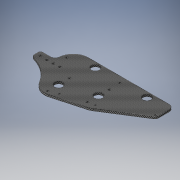
# Autodesk Inventor part: Flywheel Bracket 1
Saved by Autodesk Inventor 2019.4 (Build 234330000, 330)
## iProperties
Created: 2020-01-06
Part Number: Flywheel Bracket 1
Material: CFRP
Document SubType Name: Modeling
Designer: admin
Density: 1.43 g/cm^3
Appearance: Carbon Fiber
Mass: 143.228 g
Surface Area: 462.815 cm^2
Volume: 100.16 cm^3
Author: admin
Autodesk Inventor part; units mm, degrees
ref_plane "YZ Plane" through (0, 0, 0) normal (1, 0, 0) x (0, 1, 0)
ref_plane "XZ Plane" through (0, 0, 0) normal (0, 1, 0) x (-1, 0, 0)
ref_plane "XY Plane" through (0, 0, 0) normal (0, 0, 1) x (1, 0, 0)
sketch "Sketch1" plane through (0, 0, 0) normal (0, 1, 0) x (-1, 0, 0)
  circle A0 centre (-15.2408, 30.085) radius 9.5
  circle A1 centre (-15.2408, 30.085) radius 41.275 construction
  circle A2 centre (44.7592, 83) radius 9.5
  circle A3 centre (113.125, 107.1321) radius 9.5
  circle A4 centre (104.7592, 30.085) radius 9.5
  circle A5 centre (104.7592, 30.085) radius 41.275 construction
  line L0 (104.7592, 30.085) -> (-15.2408, 30.085) construction
  circle A6 centre (44.7592, 83) radius 32.5 construction
  circle A7 centre (113.125, 107.1321) radius 32.5 construction
  circle A8 centre (44.7592, -74.69) radius 88.9 construction
  line L1 (144.134, -74.69) -> (-106.866, -74.69) construction
  line L2 (113.125, 107.1321) -> (44.7592, 83) construction
  line L3 (44.7592, 83) -> (-15.2408, 30.085) construction
  line L4 (113.125, 107.1321) -> (104.7592, 30.085) construction
  line L5 (44.7592, 83) -> (104.7592, 30.085) construction
  line L6 (44.7592, 30.085) -> (44.7592, -74.69) construction
  line L7 (168.125, 18.085) -> (-65.2408, 18.085)
  line L8 (-65.2408, 18.085) -> (-65.2408, 58.085)
  line L9 (-65.2408, 58.085) -> (29.4431, 117.669)
  line L10 (29.4431, 117.669) -> (127.8623, 144.9403)
  line L11 (127.8623, 144.9403) -> (168.125, 80.31)
  line L12 (168.125, 80.31) -> (202.259, 80.31)
  line L13 (202.259, 80.31) -> (202.259, 60.31)
  line L14 (168.125, 18.085) -> (168.125, 60.31)
  line L15 (168.125, 60.31) -> (202.259, 60.31)
  line L16 (168.125, 80.31) -> (168.125, 60.31) construction
  circle A9 centre (44.7592, 83) radius 37.5 construction
  circle A10 centre (192.259, 70.31) radius 2.75
  line L17 (192.259, 70.31) -> (147.259, 70.31) construction
  circle A11 centre (147.259, 70.31) radius 2.75
  circle A12 centre (177.259, 70.31) radius 2.75
  circle A13 centre (162.259, 70.31) radius 2.75
  line L18 (44.7592, 57.6) -> (44.7592, 108.4) construction
  circle A14 centre (44.7592, 57.6) radius 2.75
  circle A15 centre (44.7592, 108.4) radius 2.75
  circle A16 centre (-60.2408, 55.3238) radius 2.2
  circle A17 centre (-60.2408, 55.3238) radius 5 construction
  circle A18 centre (28.7684, 105.4292) radius 2.2
  circle A19 centre (44.7592, 33.085) radius 2.2
  circle A20 centre (93.1857, 124.9549) radius 2.2
  circle A21 centre (158.125, 43.085) radius 2.2
  line L19 (113.125, 81.7321) -> (113.125, 132.5321) construction
  circle A22 centre (113.125, 81.7321) radius 2.75
  circle A23 centre (113.125, 132.5321) radius 2.75
  dimension "d67" = 19
  dimension "d68" = 82.55
  dimension "d69" = 19
  dimension "d70" = 19
  dimension "d71" = 19
  dimension "d72" = 82.55
  dimension "d73" = 65
  dimension "d74" = 65
  dimension "d75" = 120
  dimension "d76" = 177.8
  dimension "d77" = 104.775
  dimension "d78" = 80
  dimension "d79" = 80
  dimension "d80" = 77.5
  dimension "d81" = 72.5
  dimension "d82" = 12
  dimension "d83" = 50
  dimension "d85" = 75
  dimension "d86" = 20
  dimension "d87" = 34.134
  dimension "d88" = 5.5
  dimension "d90" = 5.5
  dimension "d91" = 5.5
  dimension "d93" = 15
  dimension "d95" = 5.5
  dimension "d96" = 15
  dimension "d97" = 15
  dimension "d98" = 10
  dimension "d99" = 10
  dimension "d100" = 135
  dimension "d101" = 40
  dimension "d105" = 55
  dimension "d106" = 50.8
  dimension "d107" = 5.5
  dimension "d108" = 5.5
  dimension "d112" = 4.4
  dimension "d113" = 10
  dimension "d114" = 4.4
  dimension "d115" = 4.4
  dimension "d116" = 4.4
  dimension "d117" = 4.4
  dimension "d118" = 10
  dimension "d119" = 25
  dimension "d120" = 15
  dimension "d121" = 110
  dimension "d122" = 10
  dimension "d123" = 10
  dimension "d124" = 40
  dimension "d125" = 105
  dimension "d127" = 5.5
  dimension "d128" = 5.5
  dimension "d129" = 50.8
  constraints: 41 end point, 24 centre point, 10 coincident, 6 tangent, 5 horizontal, 4 perpendicular, 3 midpoint, 3 point on line, 3 vertical, 1 parallel
  measures "d67" diameter of A0
  measures "d68" diameter of A1
  measures "d69" diameter of A2
  measures "d70" diameter of A3
  measures "d71" diameter of A4
  measures "d72" diameter of A5
  measures "d73" diameter of A6
  measures "d74" diameter of A7
  measures "d75" distance of L0.start L0.end
  measures "d76" diameter of A8
  measures "d77" distance between parallel lines of L1 L0
  measures "d78" distance of L2.end L0.end
  measures "d79" distance of L2.end L0.start
  measures "d80" distance of L2.start L0.start
  measures "d81" distance of L2.start L2.end
  measures "d82" distance from line of L7 A4.centre
  measures "d83" distance from line of A0.centre L8
  measures "d85" diameter of A9
  measures "d86" distance of L12.end L13.end
  measures "d87" distance of L11.end L12.end
  measures "d88" diameter of A10
  measures "d90" diameter of A11
  measures "d91" diameter of A12
  measures "d93" distance of A12.centre L17.start
  measures "d95" diameter of A13
  measures "d96" distance of A12.centre A13.centre
  measures "d97" distance of L17.end A13.centre
  measures "d98" distance from line of L15 L17.start
  measures "d99" distance from line of L13 L17.start
  measures "d100" distance between parallel lines of L1 L15
  measures "d101" distance of L7.end L8.end
  measures "d105" distance from line of A3.centre L14
  measures "d106" distance of L18.start L18.end
  measures "d107" diameter of A14
  measures "d108" diameter of A15
  measures "d112" diameter of A16
  measures "d113" diameter of A17
  measures "d114" diameter of A18
  measures "d115" diameter of A19
  measures "d116" diameter of A20
  measures "d117" diameter of A21
  measures "d118" distance from line of L14 A21.centre
  measures "d119" distance from line of L7 A21.centre
  measures "d120" distance from line of L7 A19.centre
  measures "d121" distance from line of L8 A19.centre
  measures "d122" distance from line of L9 A18.centre
  measures "d123" distance from line of L10 A20.centre
  measures "d124" distance from line of L11 A20.centre
  measures "d125" distance from line of L11 A18.centre
  measures "d127" diameter of A22
  measures "d128" diameter of A23
  measures "d129" distance of L19.start L19.end
extrude "Extrusion1" add sketch "Sketch1" along normal blind 5
fillet "Fillet5" radius 10 3 edges at (-168.125, 2.5, 60.31) (65.2408, 2.5, 58.085) (65.2408, 2.5, 18.085)
fillet "Fillet6" radius 37.5 1 edges at (-29.4431, 2.5, 117.669)
fillet "Fillet7" radius 5 2 edges at (-202.259, 2.5, 80.31) (-202.259, 2.5, 60.31)
fillet "Fillet8" radius 100 1 edges at (-168.125, 2.5, 80.31)
fillet "Fillet9" radius 32.5 1 edges at (-127.8623, 2.5, 144.9403)
fillet "Fillet10" radius 35 1 edges at (-168.125, 2.5, 18.085)
body "Solid1"
